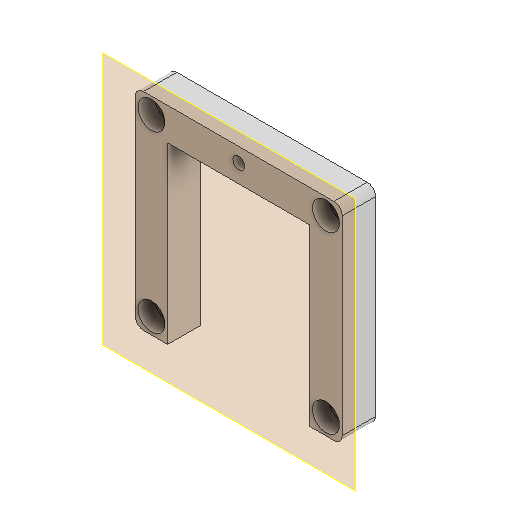
# Autodesk Inventor part: 00_Linear_Stage_NEMA11_Mount_Lid
Saved by Autodesk Inventor 2023 (Build 270158000, 158)
## iProperties
Created: 2022-02-11
Part Number: 00_Linear_Stage_NEMA11_Mount_Lid
Material: Generic
Document SubType Name: Modeling
Designer: wanghaoran
Density: 1 g/cm^3
Appearance: Default
Author: wanghaoran
Autodesk Inventor part; units mm, degrees
ref_plane "YZ Plane" through (0, 0, 0) normal (1, 0, 0) x (0, 1, 0)
ref_plane "XZ Plane" through (0, 0, 0) normal (0, 1, 0) x (-1, 0, 0)
ref_plane "XY Plane" through (0, 0, 0) normal (0, 0, 1) x (1, 0, 0)
sketch "Sketch1" plane through (0, 0, 0) normal (0, 0, 1) x (1, 0, 0)
  circle A0 centre (-21, 1.215) radius 1.4 projected
  circle A1 centre (21, 1.215) radius 1.4 projected
  arc A2 (24.9, 3.115) -> (22.9, 5.115) centre (22.9, 3.115) ccw projected
  line L0 (22.9, 5.115) -> (-22.9, 5.115) projected
  arc A3 (-22.9, 5.115) -> (-24.9, 3.115) centre (-22.9, 3.115) ccw projected
  line L1 (-24.9, 3.115) -> (-24.9, -5.115) projected
  line L2 (-24.9, -5.115) -> (-22.8395, -5.115) projected
  line L3 (24.9, -5.115) -> (24.9, 3.115) projected
  arc A4 (22.9, -44.685) -> (24.9, -42.685) centre (22.9, -42.685) ccw projected
  line L4 (24.9, -42.685) -> (24.9, -36.885) projected
  line L5 (24.9, -36.885) -> (17.1, -36.885) projected
  line L6 (17.1, -36.885) -> (17.1, -44.685) projected
  line L7 (17.1, -44.685) -> (22.9, -44.685) projected
  circle A5 centre (21, -40.785) radius 1.4 projected
  arc A6 (-24.9, -42.685) -> (-22.9, -44.685) centre (-22.9, -42.685) ccw projected
  line L8 (-22.9, -44.685) -> (-17.1, -44.685) projected
  line L9 (-17.1, -44.685) -> (-17.1, -36.885) projected
  line L10 (-17.1, -36.885) -> (-24.9, -36.885) projected
  line L11 (-24.9, -36.885) -> (-24.9, -42.685) projected
  circle A7 centre (-21, -40.785) radius 1.4 projected
  line L12 (24.9, 5.115) -> (-24.9, 5.115)
  line L13 (-24.9, 5.115) -> (-24.9, -44.685)
  line L14 (-24.9, -44.685) -> (24.9, -44.685)
  line L15 (24.9, -44.685) -> (24.9, 5.115)
  line L16 (17.1, -2.685) -> (-17.1, -2.685)
  line L17 (-17.1, -2.685) -> (-17.1, -36.885)
  line L18 (-17.1, -36.885) -> (17.1, -36.885)
  line L19 (17.1, -36.885) -> (17.1, -2.685)
  line L20 (17.1, -36.885) -> (17.1, -44.685)
  line L21 (-17.1, -36.885) -> (-17.1, -44.685)
  circle A8 centre (0, 1.415) radius 1.4 projected
  arc A9 (-18.2605, -5.115) -> (-22.8395, -5.115) centre (-20.55, -5.335) ccw projected
  arc A10 (22.8395, -5.115) -> (18.2605, -5.115) centre (20.55, -5.335) ccw projected
  circle A11 centre (14.45, 0.765) radius 2.3 projected
  circle A12 centre (-14.45, 0.765) radius 2.3 projected
  line L22 (-18.2605, -5.115) -> (18.2605, -5.115) projected
  line L23 (22.8395, -5.115) -> (24.9, -5.115) projected
  point P0 (0, 0)
  point P1 (-20.55, -5.335)
  point P2 (20.55, -5.335)
  point P3 (-20.55, -5.335)
  point P4 (20.55, -5.335)
  point P5 (-20.55, -5.335)
  point P6 (20.55, -5.335)
  dimension "d0" = 7.8
  constraints: 20 end point, 6 equal length, 2 perpendicular, 1 horizontal, 1 point on line, 3 other
  measures "d0" distance between parallel lines of L15 L19
extrude "Extrusion1" add sketch "Sketch1" along normal blind 8 contours L3 L23 A10 L22 L19 L16 L17 A9 L2 L1 A3 L0 A2 | L15 L5 L19 L22 A10 L23 | L4 A4 L7 L6 L5 | L2 A9 L22 L17 L10 L13 | L9 L8 A6 L11 L10 | A8 | A11 | A12
sketch "Sketch2" plane through (0, 0, 8) normal (0, 0, 1) x (1, 0, 0)
  circle A0 centre (0, 1.715) radius 1.4
  line L0 (22.9, 5.115) -> (-22.9, 5.115) projected
  point P0 (0, 0)
  dimension "d3" = 2.8
  dimension "d4" = 3.4
  constraints: 1 centre point
  measures "d3" diameter of A0
  measures "d4" distance from line of L0 A0.centre
extrude "Extrusion2" cut sketch "Sketch2" against normal blind 8
ref_plane "Arbeitsebene1" through (15.3065, -4.4785, 13.1) normal (0, 0, 1) x (0, 1, 0)
sketch "Skizze3" plane through (15.3065, -4.4785, 13.1) normal (0, 0, 1) x (0, 1, 0)
  line L0 (-0.7065, 32.7565) -> (-31.2065, 32.7565) projected
  arc A0 (1.2935, 30.7565) -> (-0.7065, 32.7565) centre (-0.7065, 30.7565) ccw projected
  line L1 (1.2935, 30.7565) -> (1.2935, 0.2565) projected
  arc A1 (-0.7065, -1.7435) -> (1.2935, 0.2565) centre (-0.7065, 0.2565) ccw projected
  line L2 (-0.7065, -1.7435) -> (-31.2065, -1.7435) projected
  arc A2 (-33.2065, 0.2565) -> (-31.2065, -1.7435) centre (-31.2065, 0.2565) ccw projected
  line L3 (-33.2065, 0.2565) -> (-33.2065, 30.7565) projected
  arc A3 (-31.2065, 32.7565) -> (-33.2065, 30.7565) centre (-31.2065, 30.7565) ccw projected
  line L4 (-38.9565, -9.4935) -> (-20.9565, -9.4935) projected
  arc A4 (7.0435, -9.4935) -> (9.0435, -7.4935) centre (7.0435, -7.4935) ccw projected
  line L5 (9.0435, 10.5065) -> (9.0435, -7.4935) projected
  line L6 (9.0435, 10.5065) -> (10.195, 10.5065) projected
  arc A5 (10.6845, 10.1086) -> (10.195, 10.5065) centre (10.195, 10.0065) ccw projected
  arc A6 (10.6845, 10.1086) -> (14.5435, 10.5065) centre (12.5935, 10.5065) ccw projected
  line L7 (14.5435, 10.5065) -> (14.5435, 20.6065) projected
  line L8 (9.0435, 38.5065) -> (9.0435, 20.5065) projected
  arc A7 (9.0435, 38.5065) -> (7.0435, 40.5065) centre (7.0435, 38.5065) ccw projected
  line L9 (-21.0689, 40.5065) -> (-38.9565, 40.5065) projected
  line L10 (7.0435, 40.5065) -> (-10.8565, 40.5065) projected
  arc A8 (-38.9565, 40.5065) -> (-40.9565, 38.5065) centre (-38.9565, 38.5065) ccw projected
  line L11 (-40.9565, 20.6065) -> (-40.9565, 38.5065) projected
  line L12 (-40.9565, -7.4935) -> (-40.9565, 10.3942) projected
  arc A9 (-40.9565, -7.4935) -> (-38.9565, -9.4935) centre (-38.9565, -7.4935) ccw projected
  line L13 (-20.9565, -9.4935) -> (-20.9565, -10.645) projected
  arc A10 (-21.3545, -11.1345) -> (-20.9565, -10.645) centre (-21.4565, -10.645) ccw projected
  arc A11 (-21.3545, -11.1345) -> (-20.9565, -14.9935) centre (-20.9565, -13.0435) ccw projected
  line L14 (-20.9565, -14.9935) -> (-10.8565, -14.9935) projected
  circle A12 centre (-15.9565, -5.8535) radius 1.6 projected
  circle A13 centre (5.4035, 15.5065) radius 1.6 projected
  line L15 (-21.0689, 39.3752) -> (-21.0689, 40.5065) projected
  line L16 (-40.9565, 20.6065) -> (-39.8237, 20.6065) projected
  arc A14 (-39.8237, 20.6065) -> (-39.429, 20.9412) centre (-39.8237, 21.0065) ccw projected
  arc A15 (-35.3565, 20.6065) -> (-39.429, 20.9412) centre (-37.4065, 20.6065) ccw projected
  line L17 (-35.3565, 20.6065) -> (-35.3565, 10.5065) projected
  arc A16 (-39.4194, 10.1183) -> (-35.3565, 10.5065) centre (-37.4065, 10.5065) ccw projected
  arc A17 (-39.4194, 10.1183) -> (-39.8252, 10.3942) centre (-39.7609, 10.0524) ccw projected
  line L18 (-39.8252, 10.3942) -> (-40.9565, 10.3942) projected
  arc A18 (-10.8565, -14.9935) -> (-10.5382, -11.1196) centre (-10.8565, -13.0435) ccw projected
  arc A19 (-10.9565, -10.6263) -> (-10.5382, -11.1196) centre (-10.4565, -10.6263) ccw projected
  line L19 (-10.9565, -10.6263) -> (-10.9565, -9.4935) projected
  line L20 (-10.9565, -9.4935) -> (7.0435, -9.4935) projected
  arc A20 (14.5435, 20.6065) -> (10.6696, 20.9249) centre (12.5935, 20.6065) ccw projected
  arc A21 (10.1763, 20.5065) -> (10.6696, 20.9249) centre (10.1763, 21.0065) ccw projected
  line L21 (10.1763, 20.5065) -> (9.0435, 20.5065) projected
  line L22 (-10.8565, 40.5065) -> (-10.8565, 39.3737) projected
  arc A22 (-10.8565, 39.3737) -> (-10.5218, 38.979) centre (-10.4565, 39.3737) ccw projected
  arc A23 (-10.8565, 34.9065) -> (-10.5218, 38.979) centre (-10.8565, 36.9565) ccw projected
  line L23 (-10.8565, 34.9065) -> (-20.9565, 34.9065) projected
  arc A24 (-21.3448, 38.9694) -> (-20.9565, 34.9065) centre (-20.9565, 36.9565) ccw projected
  arc A25 (-21.3448, 38.9694) -> (-21.0689, 39.3752) centre (-21.4107, 39.3109) ccw projected
  circle A26 centre (4.0435, -4.4935) radius 2.45 projected
  circle A27 centre (-1.4565, -5.2935) radius 2.3 projected
  circle A28 centre (4.8435, 1.0065) radius 2.3 projected
  circle A29 centre (4.8435, 30.0065) radius 2.3 projected
  circle A30 centre (-1.4565, 36.3065) radius 2.3 projected
  circle A31 centre (4.0435, 35.5065) radius 2.45 projected
  circle A32 centre (-36.7565, 1.0065) radius 2.3 projected
  circle A33 centre (-30.4565, -5.2935) radius 2.3 projected
  circle A34 centre (-35.9565, -4.4935) radius 2.45 projected
  circle A35 centre (-36.7565, 30.0065) radius 2.3 projected
  circle A36 centre (-30.4565, 36.3065) radius 2.3 projected
  circle A37 centre (-35.9565, 35.5065) radius 2.45 projected
  point P0 (4.4785, 15.3065)
hole "Bohrung1" [suppressed]
sketch "Skizze4" plane through (0, 0, 8) normal (0, 0, 1) x (1, 0, 0)
  circle A0 centre (0, 1.715) radius 1.4 projected
  line L0 (17.1, -2.685) -> (17.1, -44.685) projected
  line L1 (17.1, -44.685) -> (22.9, -44.685) projected
  arc A1 (22.9, -44.685) -> (24.9, -42.685) centre (22.9, -42.685) ccw projected
  line L2 (24.9, -42.685) -> (24.9, 3.115) projected
  arc A2 (24.9, 3.115) -> (22.9, 5.115) centre (22.9, 3.115) ccw projected
  line L3 (22.9, 5.115) -> (-22.9, 5.115) projected
  arc A3 (-22.9, 5.115) -> (-24.9, 3.115) centre (-22.9, 3.115) ccw projected
  line L4 (-24.9, 3.115) -> (-24.9, -42.685) projected
  arc A4 (-24.9, -42.685) -> (-22.9, -44.685) centre (-22.9, -42.685) ccw projected
  line L5 (-22.9, -44.685) -> (-17.1, -44.685) projected
  line L6 (-17.1, -44.685) -> (-17.1, -2.685) projected
  line L7 (-17.1, -2.685) -> (17.1, -2.685) projected
  circle A5 centre (-21, -40.785) radius 1.4 projected
  circle A6 centre (21, -40.785) radius 1.4 projected
  circle A7 centre (-21, 1.215) radius 1.4 projected
  circle A8 centre (21, 1.215) radius 1.4 projected
  point P0 (0, 0)
hole "Bohrung2" at (-21, 1.215, 8) at (21, 1.215, 8) at (21, -40.785, 8) at (-21, -40.785, 8) direction (0, 0, -1) diameter 3 end through all counterbore diameter 6.5 counterbore depth 4
body "Solid1"
